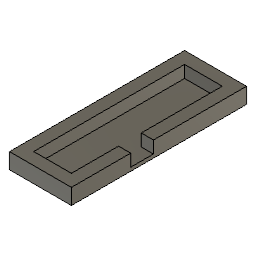
Hackpad (Autodesk Fusion 360 design; units mm, degrees)
part number: 2026-04-13-16-54-27-480
Autodesk Fusion 360 part; units mm, degrees
sketch "Sketch1" plane through (0, 0, 0) normal (0, 0, 1) x (1, 0, 0)
  line L0 (0, 0) -> (51, 0)
  line L1 (51, 0) -> (51, 144)
  line L2 (51, 144) -> (0, 144)
  line L3 (0, 144) -> (0, 0)
  line L4 (10, 10) -> (41, 10)
  line L5 (41, 10) -> (41, 134)
  line L6 (41, 134) -> (10, 134)
  line L7 (10, 134) -> (10, 10)
  dimension "d1" = 51
  dimension "d2" = 144
  dimension "d5" = 31
  dimension "d6" = 124
  constraint horizontal L0
  constraint vertical L1
  constraint horizontal L2
  constraint vertical L3
  constraint coincident L0.start L3.end
  constraint horizontal L4
  constraint vertical L5
  constraint horizontal L6
  constraint vertical L7
  measures "d1" distance of L0.start L0.end
  measures "d2" distance of L0.start L2.end
  measures "d5" distance of L4.start L4.end
  measures "d6" distance of L4.start L6.end
extrude "Extrude1" add sketch "Sketch1" along normal blind 13
sketch "Sketch2" plane through (0, 0, 0) normal (0, 0, -1) x (1, 0, 0)
  line L0 (10, -134) -> (10, -10)
  line L1 (10, -10) -> (41, -10)
  line L2 (41, -10) -> (41, -134)
  line L3 (41, -134) -> (10, -134)
  line L4 (0, 0) -> (0, -144)
  line L5 (0, -144) -> (51, -144)
  line L6 (51, -144) -> (51, 0)
  line L7 (51, 0) -> (0, 0)
  line L8 (41, -134) -> (10, -134)
  line L9 (10, -134) -> (10, -10)
  line L10 (10, -10) -> (41, -10)
  line L11 (41, -10) -> (41, -134)
  constraint horizontal L8
  constraint vertical L9
  constraint horizontal L10
  constraint vertical L11
  constraint coincident L0.end L1.start
  constraint coincident L2.end L3.start
extrude "Extrude2" add sketch "Sketch2" against normal blind 3 contours L0 L1 L2 L3 L8 L9 L10 L11
sketch "Sketch3" plane through (0, 0, 13) normal (0, 0, 1) x (-1, 0, 0)
  line L0 (-10, -10) -> (-10, -134)
  line L1 (-10, -134) -> (-41, -134)
  line L2 (-41, -134) -> (-41, -10)
  line L3 (-41, -10) -> (-10, -10)
  line L4 (0, -144) -> (0, 0)
  line L5 (0, 0) -> (-51, 0)
  line L6 (-51, 0) -> (-51, -144)
  line L7 (-51, -144) -> (0, -144)
  line L8 (-41, -48.7) -> (-41, -67.4)
  line L9 (-41, -48.7) -> (-51, -48.7)
  line L10 (-51, -48.7) -> (-51, -67.4)
  line L11 (-51, -67.4) -> (-41, -67.4)
  line L12 (-41, -67.4) -> (-41, -48.7)
  dimension "d11" = 38.7
  dimension "d12" = 18.7
  dimension "d13" = 18.7
  constraint parallel L2 L8
  constraint horizontal L9
  constraint vertical L10
  constraint horizontal L11
  constraint vertical L12
  measures "d11" distance of L2.end L8.start
  measures "d12" distance of L8.start L8.end
  measures "d13" distance of L8.start L8.end
extrude "Extrude3" cut sketch "Sketch3" against normal blind 10 contours L2 L6 L8 L9 L10 L11 L12
